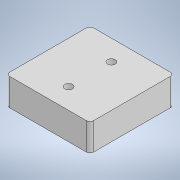
# Autodesk Inventor part: 31_Y-Motor_cable_holder
Saved by Autodesk Inventor 2022 (Build 260153000, 153)
## iProperties
Created: 2023-01-15
Part Number: 31_Y-Motor_cable_holder
Material: Generic
Document SubType Name: Modeling
Designer: Max
Density: 1 g/cm^3
Appearance: Default
Author: Max
Autodesk Inventor part; units mm, degrees
ref_plane "YZ Plane" through (0, 0, 0) normal (1, 0, 0) x (0, 1, 0)
ref_plane "XZ Plane" through (0, 0, 0) normal (0, 1, 0) x (-1, 0, 0)
ref_plane "XY Plane" through (0, 0, 0) normal (0, 0, 1) x (1, 0, 0)
sketch "Sketch1" plane through (0, 0, 0) normal (0, 1, 0) x (-1, 0, 0)
  line L0 (21.55, 21.55) -> (-21.55, 21.55)
  line L1 (-21.55, 21.55) -> (-21.55, -21.55)
  line L2 (-21.55, -21.55) -> (21.55, -21.55)
  line L3 (21.55, -21.55) -> (21.55, 21.55)
  line L4 (21.55, 21.55) -> (-21.55, -21.55) construction
  line L5 (-21.55, 21.55) -> (21.55, -21.55) construction
  point P0 (0, 0)
  dimension "d0" = 43.1
  dimension "d1" = 43.1
  constraints: 12 end point, 2 midpoint, 2 parallel, 1 horizontal, 1 perpendicular
  measures "d0" distance of L2.end L1.end
  measures "d1" distance between parallel lines of L0 L2
extrude "Extrusion1" add sketch "Sketch1" along normal blind 14
sketch "Sketch2" plane through (0, 0, 0) normal (0, -1, 0) x (1, 0, 0)
  line L0 (-20.05, 20.05) -> (20.05, 20.05)
  line L1 (20.05, 20.05) -> (20.05, -20.05)
  line L2 (20.05, -20.05) -> (-20.05, -20.05)
  line L3 (-20.05, -20.05) -> (-20.05, 20.05)
  line L4 (-20.05, 20.05) -> (20.05, -20.05) construction
  line L5 (20.05, 20.05) -> (-20.05, -20.05) construction
  point P0 (0, 0)
  dimension "d4" = 40.1
  dimension "d5" = 40.1
  constraints: 12 end point, 2 midpoint, 2 parallel, 1 horizontal, 1 perpendicular
  measures "d4" distance of L1.end L2.end
  measures "d5" distance between parallel lines of L0 L2
extrude "Extrusion2" cut sketch "Sketch2" against normal blind 8
fillet "Fillet1" radius 2 4 edges at (-21.55, 7, 21.55) (21.55, 7, 21.55) (21.55, 7, -21.55) (-21.55, 7, -21.55)
sketch "Sketch3" plane through (0, 14, 0) normal (0, 1, 0) x (1, 0, 0)
  line L0 (0, 30.17) -> (0, -30.17) projected
  circle A0 centre (0, -11) radius 2
  circle A1 centre (0, 11) radius 2
  line L1 (30.17, 0) -> (-30.17, 0) projected
  point P0 (0, 0)
  dimension "d9" = 4
  dimension "d10" = 22
  constraints: 2 centre point, 2 point on line, 1 equal radius, 1 other
  measures "d9" diameter of A0
  measures "d10" distance of A1.centre A0.centre
extrude "Extrusion3" cut sketch "Sketch3" against normal through all
equation "\"d1\" = d0"
equation "\"d5\" = d4"
body "Solid1"
